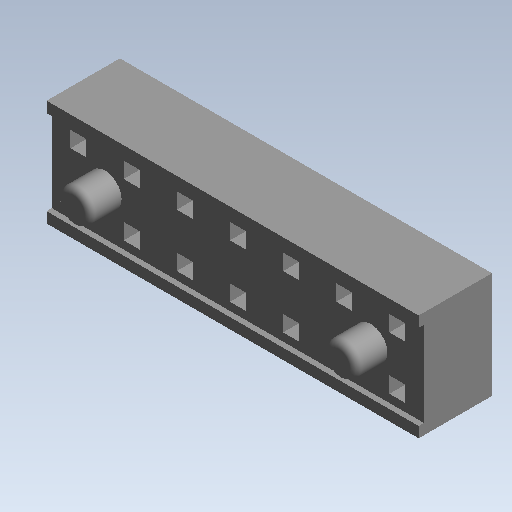
# Autodesk Inventor part: HLE-107-02-DV-A_socket
Saved by Autodesk Inventor 2021 (Build 250183000, 183)
## iProperties
Part Number: HLE-107-02-DV-A_socket
Material: Generic
Catalog Web Link: www.cadenas.de
Description: HLE--Socket
Vendor: SAMTEC
Document SubType Name: Modeling
Designer: partserver
Manufacturer: SAMTEC
Mass: 0.270296 g
Surface Area: 5.28692 cm^2
Volume: 0.270296 cm^3
Density: 1 g/cm^3
Appearance: PSOLRGB-175-175-175
Category: PARTsolutions
Company: SAMTEC
PSOL_IDENT_0: {$CADENAS_DATA\23d-libs\samtec\modelling\hle\parts\hle_socket.prj},196 {VTYP=3D},{NB=HLE-107-02-DV-A
PSOL_IDENT_1: _socket},{LINA=HLE-107-02-DV-A_socket},{NN=HLE-},{DATE=08.04.2016 05:41:54},{GEOMDATE=07.04.2016 12:
PSOL_IDENT_2: 48:00},{VERSION=},{LINEID=10},{WBVAR=POS,AOPT,LCOPT},{WBNUMERIC=}  {NB=HLE-107-02-DV-A_socket},{LINA=
PSOL_IDENT_3: HLE-107-02-DV-A_socket},{KT=DUMMY},{PN=HLE-107-02-DV-A},{SERIES=HLE},{POSALG=  '02' , '-02' , '03' ,
PSOL_IDENT_4: '-03' , '04' , '-04' , '05' , '-05' , '06' , '-06' , '07' , '-07' , '08' , '-08' , '09' , '-09' , '
PSOL_IDENT_5: 10' , '-10' , '11' , '-11' , '12' , '-12' , '13' , '-13' , '14' , '-14' , '15' , '-15' , '16' , '-16'
PSOL_IDENT_6: , '17' , '-17' , '18' , '-18' , '19' , '-19' , '20' , '-20' , '21' , '-21' , '22' , '-22' , '23' , '
PSOL_IDENT_7: -23' , '24' , '-24' , '25' , '-25' , '26' , '-26' , '27' , '-27' , '28' , '-28' , '29' , '-29' , '30'
PSOL_IDENT_8: , '-30' , '31' , '-31' , '32' , '-32' , '33' , '-33' , '34' , '-34' , '35' , '-35' , '36' , '-36' ,
PSOL_IDENT_9: '37' , '-37' , '38' , '-38' , '39' , '-39' , '40' , '-40'  , '41' , '-41' , '42' , '-42' , '43' , '
PSOL_IDENT_10: -43' , '44' , '-44' , '45' , '-45' , '46' , '-46' , '47' , '-47' , '48' , '-48' , '49' , '-49' , '50'
PSOL_IDENT_11: , '-50'   },{POS=07},{LSALG=  '02' , '-02 - Surface Mount'  },{LS=02 - Surface Mount},{ROPTALG=   '
PSOL_IDENT_12: DV' , '-DV - Double Vertical'  },{ROPT=DV},{AOPTALG=    ''  , 'Not Selected'  ,  'A' , '-A - Alignme
PSOL_IDENT_13: nt Pins'   },{AOPT=A},{LCOPTALG= '' , 'Not Available' },{LCOPT=},{B=0.138},{PINS=7},{W=0.2000},{LC=0
PSOL_IDENT_14: .050},{L=0.70000},{PINW=0.020},{PITCH=0.1000},{PITCH2=0.1000},{AOPTPN=-A},{LCPN=}
NB: HLE-107-02-DV-A_socket
NN: HLE-
NT: Socket
NBSYN: $PN._socket
LINA: HLE-107-02-DV-A_socket
CATALOG: Samtec
PN: HLE-107-02-DV-A
SERIES: HLE
POS: -07
LS: 02 - Surface Mount
ROPT: DV
AOPT: -A - Alignment Pins
LCOPT: Not Available
B: 0.138
W: 0.2
LC: 0.05
L: 0.7
PINW: 0.02
PITCH: 0.1
PITCH2: 0.1
SUPPLIER: SAMTEC
ARTICLENO: HLE-107-02-DV-A_socket
BOMINFO: HLE-107-02-DV-A_socket
CREATOR: CADENAS GmbH
Title: HLE-107-02-DV-A_socket
Author: Cadenas PARTsolutions
Comments: Socket
Autodesk Inventor part; units mm, degrees
ref_plane "YZ Plane" through (0, 0, 0) normal (1, 0, 0) x (0, 1, 0)
ref_plane "XZ Plane" through (0, 0, 0) normal (0, 1, 0) x (-1, 0, 0)
ref_plane "XY Plane" through (0, 0, 0) normal (0, 0, 1) x (1, 0, 0)
sketch "Sketch_1" plane through (0, 0, 0) normal (0, 1, 0) x (1, 0, 0)
  line L0 (-8.89, 2.54) -> (-8.89, -2.54)
  line L1 (-8.89, -2.54) -> (8.89, -2.54)
  line L2 (8.89, -2.54) -> (8.89, 2.54)
  line L3 (8.89, 2.54) -> (-8.89, 2.54)
  line L4 (7.239, -0.889) -> (7.239, -1.651)
  line L5 (7.239, -1.651) -> (8.001, -1.651)
  line L6 (8.001, -1.651) -> (8.001, -0.889)
  line L7 (8.001, -0.889) -> (7.239, -0.889)
  line L8 (7.239, 1.651) -> (7.239, 0.889)
  line L9 (7.239, 0.889) -> (8.001, 0.889)
  line L10 (8.001, 0.889) -> (8.001, 1.651)
  line L11 (8.001, 1.651) -> (7.239, 1.651)
  line L12 (4.699, -0.889) -> (4.699, -1.651)
  line L13 (4.699, -1.651) -> (5.461, -1.651)
  line L14 (5.461, -1.651) -> (5.461, -0.889)
  line L15 (5.461, -0.889) -> (4.699, -0.889)
  line L16 (4.699, 1.651) -> (4.699, 0.889)
  line L17 (4.699, 0.889) -> (5.461, 0.889)
  line L18 (5.461, 0.889) -> (5.461, 1.651)
  line L19 (5.461, 1.651) -> (4.699, 1.651)
  line L20 (2.159, -0.889) -> (2.159, -1.651)
  line L21 (2.159, -1.651) -> (2.921, -1.651)
  line L22 (2.921, -1.651) -> (2.921, -0.889)
  line L23 (2.921, -0.889) -> (2.159, -0.889)
  line L24 (2.159, 1.651) -> (2.159, 0.889)
  line L25 (2.159, 0.889) -> (2.921, 0.889)
  line L26 (2.921, 0.889) -> (2.921, 1.651)
  line L27 (2.921, 1.651) -> (2.159, 1.651)
  line L28 (-0.381, -0.889) -> (-0.381, -1.651)
  line L29 (-0.381, -1.651) -> (0.381, -1.651)
  line L30 (0.381, -1.651) -> (0.381, -0.889)
  line L31 (0.381, -0.889) -> (-0.381, -0.889)
  line L32 (-0.381, 1.651) -> (-0.381, 0.889)
  line L33 (-0.381, 0.889) -> (0.381, 0.889)
  line L34 (0.381, 0.889) -> (0.381, 1.651)
  line L35 (0.381, 1.651) -> (-0.381, 1.651)
  line L36 (-2.921, -0.889) -> (-2.921, -1.651)
  line L37 (-2.921, -1.651) -> (-2.159, -1.651)
  line L38 (-2.159, -1.651) -> (-2.159, -0.889)
  line L39 (-2.159, -0.889) -> (-2.921, -0.889)
  line L40 (-2.921, 1.651) -> (-2.921, 0.889)
  line L41 (-2.921, 0.889) -> (-2.159, 0.889)
  line L42 (-2.159, 0.889) -> (-2.159, 1.651)
  line L43 (-2.159, 1.651) -> (-2.921, 1.651)
  line L44 (-5.461, -0.889) -> (-5.461, -1.651)
  line L45 (-5.461, -1.651) -> (-4.699, -1.651)
  line L46 (-4.699, -1.651) -> (-4.699, -0.889)
  line L47 (-4.699, -0.889) -> (-5.461, -0.889)
  line L48 (-5.461, 1.651) -> (-5.461, 0.889)
  line L49 (-5.461, 0.889) -> (-4.699, 0.889)
  line L50 (-4.699, 0.889) -> (-4.699, 1.651)
  line L51 (-4.699, 1.651) -> (-5.461, 1.651)
  line L52 (-8.001, -0.889) -> (-8.001, -1.651)
  line L53 (-8.001, -1.651) -> (-7.239, -1.651)
  line L54 (-7.239, -1.651) -> (-7.239, -0.889)
  line L55 (-7.239, -0.889) -> (-8.001, -0.889)
  line L56 (-8.001, 1.651) -> (-8.001, 0.889)
  line L57 (-8.001, 0.889) -> (-7.239, 0.889)
  line L58 (-7.239, 0.889) -> (-7.239, 1.651)
  line L59 (-7.239, 1.651) -> (-8.001, 1.651)
  constraints: 120 end point
extrude "Extrusion1" add sketch "Sketch_1" along normal blind 3.5052
sketch "Sketch_4" plane through (0, 0, 0) normal (1, 0, 0) x (0, 1, 0)
  line L0 (0.254, 2.032) -> (0, 2.032)
  line L1 (0, 2.032) -> (0, -2.032)
  line L2 (0, -2.032) -> (0.254, -2.032)
  line L3 (0.254, -2.032) -> (0.254, 2.032)
  constraints: 8 end point
extrude "Extrusion2" cut sketch "Sketch_4" along normal mid plane 17.78
sketch "Sketch_9" plane through (0, 0, 0) normal (0, 0, 1) x (1, 0, 0)
  line L0 (6.35, -1.27) -> (6.35, 0.635)
  line L1 (6.35, 0.635) -> (7.1437, 0.635)
  line L2 (7.1437, 0.635) -> (7.1437, -0.9842)
  arc A0 (6.858, -1.27) -> (7.1437, -0.9842) centre (6.858, -0.9843) ccw
  line L3 (6.858, -1.27) -> (6.35, -1.27)
  line L4 (6.35, -1.27) -> (6.35, 0.635)
  constraints: 10 end point, 2 point on circle, 1 centre point
revolve "Revolution1" add sketch "Sketch_9" angle 360 about axis through (6.35, -1.27, 0) along (0, -1, 0)
sketch "Sketch_10" plane through (0, 0, 0) normal (0, 0, 1) x (1, 0, 0)
  line L0 (-6.35, -1.27) -> (-6.35, 0.635)
  line L1 (-6.35, 0.635) -> (-5.5563, 0.635)
  line L2 (-5.5563, 0.635) -> (-5.5563, -0.9525)
  arc A0 (-5.8738, -1.27) -> (-5.5563, -0.9525) centre (-5.8738, -0.9525) ccw
  line L3 (-5.8738, -1.27) -> (-6.35, -1.27)
  line L4 (-6.35, -1.27) -> (-6.35, 0.635)
  constraints: 10 end point, 2 point on circle, 1 centre point
revolve "Revolution2" add sketch "Sketch_10" angle 360 about axis through (-6.35, -1.27, 0) along (0, -1, 0)
sketch "Sketch_11" plane through (0, 3.5052, 0) normal (0, 1, 0) x (1, 0, 0)
  line L0 (-6.5405, 1.27) -> (-6.5405, -1.27)
  line L1 (-6.5405, -1.27) -> (-6.1595, -1.27)
  line L2 (-6.1595, -1.27) -> (-6.1595, 1.27)
  line L3 (-6.1595, 1.27) -> (-6.5405, 1.27)
  constraints: 8 end point
extrude "Extrusion3" cut sketch "Sketch_11" against normal blind 1.27
pattern_linear "Rectangular Pattern1" count 6 spacing 2.54 along (1, 0, 0) of "Extrusion3"
ref_plane "socket_to_dummy_XY" through (0, 0, 0) normal (0, -1, 0) x (1, 0, 0)
ref_plane "socket_to_dummy_YZ" through (0, 0, 0) normal (1, 0, 0) x (0, 0, 1)
ref_plane "socket_to_dummy_ZX" through (0, 0, 0) normal (0, 0, 1) x (0, -1, 0)
ref_plane "socket_to_pad_XY" through (0, 3.5052, 0) normal (0, 1, 0) x (1, 0, 0)
ref_plane "socket_to_pad_YZ" through (0, 3.5052, 0) normal (1, 0, 0) x (0, 0, -1)
ref_plane "socket_to_pad_ZX" through (0, 3.5052, 0) normal (0, 0, -1) x (0, 1, 0)
body "Solid1"
